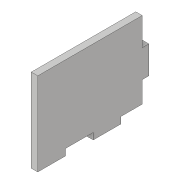
# Autodesk Inventor part: side1
Saved by Autodesk Inventor 2017 (Build 210142000, 142)
## iProperties
Created: 2019-05-21
Part Number: side1
Material: Generic
Document SubType Name: Modeling
Designer: markg
Density: 1 g/cm^3
Appearance: Default
Author: markg
Autodesk Inventor part; units mm, degrees
ref_plane "YZ Plane" through (0, 0, 0) normal (1, 0, 0) x (0, 1, 0)
ref_plane "XZ Plane" through (0, 0, 0) normal (0, 1, 0) x (-1, 0, 0)
ref_plane "XY Plane" through (0, 0, 0) normal (0, 0, 1) x (1, 0, 0)
sketch "Sketch1" plane through (0, 0, 0) normal (1, 0, 0) x (0, 1, 0)
  line L0 (-19.05, 25.4) -> (19.05, 25.4)
  line L1 (19.05, 25.4) -> (19.05, -25.4)
  line L2 (19.05, -25.4) -> (-19.05, -25.4)
  line L3 (-19.05, -25.4) -> (-19.05, 25.4)
  line L4 (-19.05, 25.4) -> (19.05, -25.4) construction
  line L5 (19.05, 25.4) -> (-19.05, -25.4) construction
  point P0 (0, 0)
  dimension "d0" = 38.1
  dimension "d1" = 50.8
  constraints: 12 end point, 2 midpoint, 2 parallel, 1 horizontal, 1 perpendicular
  measures "d0" distance of L1.end L2.end
  measures "d1" distance of L0.end L1.end
extrude "Extrusion1" add sketch "Sketch1" along normal blind 2.9718
sketch "Sketch2" plane through (2.9718, 0, 0) normal (1, 0, 0) x (0, 0, -1)
  line L0 (-25.4, -19.05) -> (25.4, -19.05) projected
  line L1 (25.4, -19.05) -> (12.7, -19.05)
  line L2 (12.7, -19.05) -> (12.7, -16.0782)
  line L3 (12.7, -16.0782) -> (25.4, -16.0782)
  line L4 (25.4, -16.0782) -> (25.4, -19.05)
  line L5 (0, -19.05) -> (-12.7, -19.05)
  line L6 (-12.7, -19.05) -> (-12.7, -16.0782)
  line L7 (-12.7, -16.0782) -> (0, -16.0782)
  line L8 (0, -16.0782) -> (0, -19.05)
  point P0 (0, 0)
  dimension "d4" = 12.7
  dimension "d5" = 2.9718
  dimension "d6" = 12.7
  constraints: 16 end point, 4 parallel, 2 horizontal, 2 perpendicular, 1 midpoint, 1 point on line
  measures "d4" distance of L2.end L3.end
  measures "d5" distance of L1.end L2.end
  measures "d6" distance of L6.end L7.end
extrude "Extrusion2" cut sketch "Sketch2" against normal blind 2.9718
sketch "Sketch3" plane through (2.9718, 0, 0) normal (1, 0, 0) x (0, 0, -1)
  line L0 (25.4, -19.05) -> (22.4282, -19.05)
  line L1 (22.4282, -19.05) -> (22.4282, -6.35)
  line L2 (22.4282, -6.35) -> (25.4, -6.35)
  line L3 (25.4, -6.35) -> (25.4, -19.05)
  line L4 (0, -19.05) -> (12.7, -19.05) projected
  line L5 (25.4, -16.0782) -> (25.4, 19.05) projected
  line L6 (25.4, 6.35) -> (22.4282, 6.35)
  line L7 (22.4282, 6.35) -> (22.4282, 19.05)
  line L8 (22.4282, 19.05) -> (25.4, 19.05)
  line L9 (25.4, 19.05) -> (25.4, 6.35)
  point P0 (0, 0)
  point P1 (25.4, 9.3218)
  dimension "d9" = 0
  dimension "d10" = 0
  dimension "d11" = 12.7
  dimension "d12" = 2.9718
  dimension "d15" = 25.4
  constraints: 16 end point, 2 parallel, 1 collinear, 1 horizontal, 1 perpendicular, 1 vertical, 8 other
  measures "d9" distance between parallel lines of L4 L0
  measures "d10" distance between parallel lines of L5 L3
  measures "d11" distance of L0.end L1.end
  measures "d12" distance of L1.end L2.end
  measures "d15" distance of L0.start L6.start
extrude "Extrusion3" cut sketch "Sketch3" against normal blind 25.4
body "Solid1"
